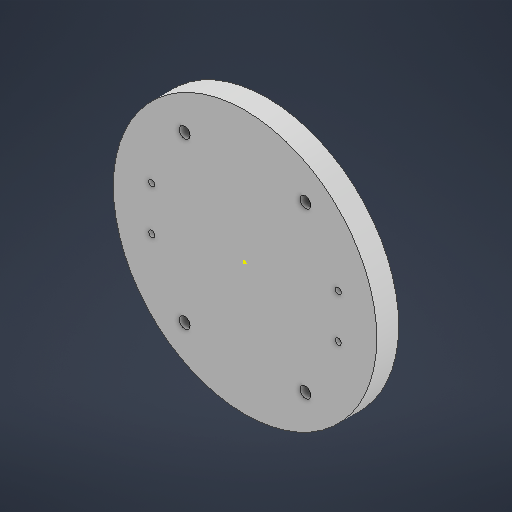
# Autodesk Inventor part: TABAN base
Saved by Autodesk Inventor 2026.1 (Build 301233020, 233B)
## iProperties
Created: 2026-04-18
Part Number: TABAN base
Material: Generic
Document SubType Name: Modeling
Designer: kadir
Density: 1 g/cm^3
Appearance: Default
Author: kadir
Autodesk Inventor part; units mm, degrees
ref_plane "YZ Plane" through (0, 0, 0) normal (1, 0, 0) x (0, 1, 0)
ref_plane "XZ Plane" through (0, 0, 0) normal (0, 1, 0) x (-1, 0, 0)
ref_plane "XY Plane" through (0, 0, 0) normal (0, 0, 1) x (1, 0, 0)
sketch "Sketch1" plane through (0, 0, 0) normal (0, 0, 1) x (1, 0, 0)
  circle A0 centre (0, 0) radius 60
  line L0 (0, 11.7433) -> (0, -11.8444)
  line L1 (-60, 0) -> (60, 0)
  circle A1 centre (-42.4915, 10) radius 1.4
  circle A2 centre (-42.4915, -10) radius 1.4
  circle A3 centre (42.4915, 10) radius 1.4
  circle A4 centre (42.4915, -10) radius 1.4
  circle A5 centre (-27.5, 37.5) radius 2.5
  circle A6 centre (-27.5, -37.5) radius 2.5
  circle A7 centre (27.5, 37.5) radius 2.5
  circle A8 centre (27.5, -37.5) radius 2.5
  point P0 (0, -0.0505)
  dimension "d0" = 2.8
  dimension "d1" = 120
  dimension "d2" = 20
  dimension "d3" = 84.983
  dimension "d4" = 5
  dimension "d5" = 55
  dimension "d6" = 75
  constraints: 9 centre point, 6 symmetric about line, 4 end point, 2 point on circle, 1 coincident, 1 horizontal, 1 midpoint, 1 vertical, 1 vertical alignment, 6 other
  measures "d0" diameter of A1
  measures "d1" diameter of A0
  measures "d2" diameter of A1.centre L1
  measures "d3" distance of A3.centre A1.centre
  measures "d4" diameter of A5
  measures "d5" diameter of A5.centre L0
  measures "d6" distance of A6.centre A5.centre
extrude "Extrusion1" add sketch "Sketch1" along normal blind 10
sketch "Sketch2" plane through (0, 0, 10) normal (0, 0, 1) x (1, 0, 0)
  point P0 (0, 0)
body "Solid1"
